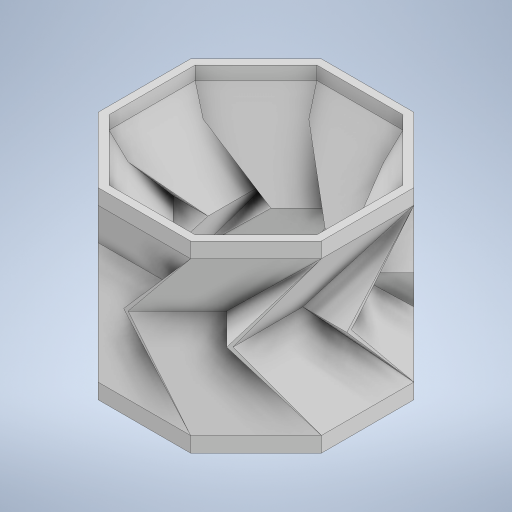
# Autodesk Inventor part: 팔각형 OV-PAM 층 한개
Saved by Autodesk Inventor 2024 (Build 280153000, 153)
## iProperties
Created: 2023-06-16
Part Number: 팔각형 OV-PAM 층 한개
Material: 일반
Document SubType Name: Modeling
Designer: jsw
Density: 1 g/cm^3
Appearance: 기본값
Author: jsw
Autodesk Inventor part; units mm, degrees
ref_plane "YZ Plane" through (0, 0, 0) normal (1, 0, 0) x (0, 1, 0)
ref_plane "XZ Plane" through (0, 0, 0) normal (0, 1, 0) x (-1, 0, 0)
ref_plane "XY Plane" through (0, 0, 0) normal (0, 0, 1) x (1, 0, 0)
sketch "스케치1" plane through (0, 0, 0) normal (0, 1, 0) x (-1, 0, 0)
  line L0 (-8.148, 3.375) -> (-3.375, 8.148)
  line L1 (-3.375, 8.148) -> (3.375, 8.148)
  line L2 (3.375, 8.148) -> (8.148, 3.375)
  line L3 (8.148, 3.375) -> (8.148, -3.375)
  line L4 (8.148, -3.375) -> (3.375, -8.148)
  line L5 (3.375, -8.148) -> (-3.375, -8.148)
  line L6 (-3.375, -8.148) -> (-8.148, -3.375)
  line L7 (-8.148, -3.375) -> (-8.148, 3.375)
  line L8 (-3.6235, 8.748) -> (3.6235, 8.748)
  line L9 (3.6235, 8.748) -> (8.748, 3.6235)
  line L10 (8.748, 3.6235) -> (8.748, -3.6235)
  line L11 (8.748, -3.6235) -> (3.6235, -8.748)
  line L12 (3.6235, -8.748) -> (-3.6235, -8.748)
  line L13 (-3.6235, -8.748) -> (-8.748, -3.6235)
  line L14 (-8.748, -3.6235) -> (-8.748, 3.6235)
  line L15 (-8.748, 3.6235) -> (-3.6235, 8.748)
  point P0 (0, 0)
  point P1 (0, 0)
  point P2 (0, 0)
  dimension "d0" = 6.75
  dimension "d2" = 0.6
  constraints: 32 end point, 2 coincident, 2 horizontal, 34 other
  measures "d0" distance of L0.end L1.end
  measures "d2" distance between parallel lines of L10 L3
extrude "돌출2" add sketch "스케치1" along normal blind 6 contours L0 L1 L2 L3 L4 L5 L6 L7 | L8 L9 L10 L11 L12 L13 L14 L15
ref_plane "작업 평면2" through (8.748, 0, 3.6235) normal (-0.8660254, -0.5, 0) x (0, 0, -1)
sketch "스케치3" plane through (8.748, 0, 3.6235) normal (1, 0, 0) x (0, 0, -1)
  line L0 (0, 0) -> (0, 6) projected
  line L1 (0, 6) -> (7.2471, 6) projected
  line L2 (0, 0) -> (7.2471, 0)
  line L3 (7.2471, 0) -> (7.2471, 6)
  line L4 (7.2471, 6) -> (0, 6)
  line L5 (0, 6) -> (0, 0)
  line L6 (0, 6) -> (-3.6524, 6)
  line L7 (-5.1244, 6) -> (0, 6) projected
  line L8 (0, 0) -> (-3.6524, 6)
  line L9 (7.2471, 6) -> (3.6235, 6)
  line L10 (7.2471, 0) -> (2, 6)
  point P0 (3.6235, 0)
  point P1 (3.6235, 6)
  point P2 (-1.4, 6)
  point P3 (2, 6)
  dimension "d17" = 121.33
  dimension "d55" = 2
  constraints: 16 end point, 6 midpoint, 2 parallel, 2 point on line, 1 horizontal, 1 perpendicular
  measures "d17" angle of L8 L2
  measures "d55" distance of L0.end L10.end
extrude "돌출4" cut sketch "스케치3" against normal up to surface contours L8 L6 L0 | L0 L1 L10 L2 surface through (8.748, 0, 3.6235) normal (-0.8660254, -0.5, 0)
pattern_circular "원형 패턴1" count 8 over 360 about axis through (0, -10, 0) along (0, 1, 0) of "돌출4"
mirror "미러5" about plane through (0, 6, 0) normal (0, 1, 0) of "돌출2", "돌출4", "원형 패턴1"
sketch "스케치9" plane through (-3.6235, 12, -8.748) normal (0, 1, 0) x (1, 0, 0)
  line L0 (12.3715, -12.3715) -> (12.3715, -5.1244) projected
  line L1 (12.3715, -5.1244) -> (7.2471, 0) projected
  line L2 (7.2471, 0) -> (0, 0) projected
  line L3 (0, 0) -> (-5.1244, -5.1244) projected
  line L4 (-5.1244, -5.1244) -> (-5.1244, -12.3715) projected
  line L5 (-5.1244, -12.3715) -> (0, -17.4959) projected
  line L6 (0, -17.4959) -> (7.2471, -17.4959) projected
  line L7 (7.2471, -17.4959) -> (12.3715, -12.3715) projected
  point P0 (3.6235, -8.748)
extrude "돌출8" add sketch "스케치9" along normal blind 1.2
sketch "스케치10" plane through (0, 0, 0) normal (0, -1, 0) x (1, 0, 0)
  line L0 (8.748, 3.6235) -> (8.748, -3.6235) projected
  line L1 (3.6235, 8.748) -> (8.748, 3.6235) projected
  line L2 (-3.6235, 8.748) -> (3.6235, 8.748) projected
  line L3 (-8.748, 3.6235) -> (-3.6235, 8.748) projected
  line L4 (-8.748, -3.6235) -> (-8.748, 3.6235) projected
  line L5 (-3.6235, -8.748) -> (-8.748, -3.6235) projected
  line L6 (3.6235, -8.748) -> (-3.6235, -8.748) projected
  line L7 (8.748, -3.6235) -> (3.6235, -8.748) projected
  point P0 (0, 0)
extrude "돌출9" add sketch "스케치10" along normal blind 1.2
shell "쉘6" thickness 0.6 removed faces 2 at (-0.5003, 13.2, 1.2078) at (1.2078, -1.2, -2.916)
